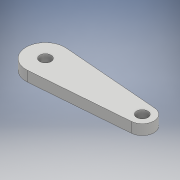
# Autodesk Inventor part: tipper_link_D_support
Saved by Autodesk Inventor 2017 (Build 210142000, 142)
## iProperties
Created: 2017-07-15
Part Number: tipper_link_D_support
Material: Generic
Document SubType Name: Modeling
Designer: Nic
Density: 1 g/cm^3
Appearance: Default
Author: Nic
Autodesk Inventor part; units mm, degrees
ref_plane "YZ Plane" through (0, 0, 0) normal (1, 0, 0) x (0, 1, 0)
ref_plane "XZ Plane" through (0, 0, 0) normal (0, 1, 0) x (-1, 0, 0)
ref_plane "XY Plane" through (0, 0, 0) normal (0, 0, 1) x (1, 0, 0)
sketch "Sketch1" plane through (0, 0, 0) normal (0, 0, 1) x (1, 0, 0)
  circle A0 centre (0, 0) radius 1.75
  line L0 (0.48, 5.9808) -> (30.288, 3.5885)
  arc A1 (30.288, -3.5885) -> (30.288, 3.5885) centre (30, 0) ccw
  line L1 (30.288, -3.5885) -> (0.48, -5.9808)
  arc A2 (0.48, 5.9808) -> (0.48, -5.9808) centre (0, 0) ccw
  circle A3 centre (30, 0) radius 1.75
  dimension "d0" = 3.5
  dimension "d1" = 6
  dimension "d2" = 30
  dimension "d9" = 3.5
  dimension "d10" = 3.6
  constraints: 4 centre point, 4 end point, 4 point on circle, 4 tangent, 2 coincident, 1 concentric, 1 horizontal alignment
  measures "d0" diameter of A0
  measures "d1" radius of A2
  measures "d2" distance of A1.centre point (0, 0)
  measures "d9" diameter of A3
  measures "d10" radius of A1
extrude "Extrusion1" add sketch "Sketch1" along normal blind 3.175
body "Solid1"
